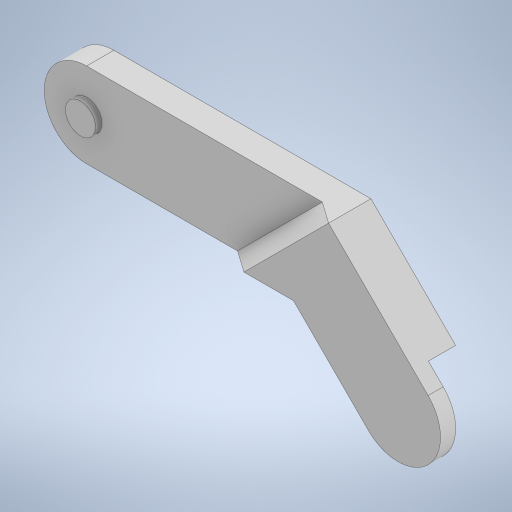
# Autodesk Inventor part: arm 1 leftt
Saved by Autodesk Inventor 2023 (Build 270158000, 158)
## iProperties
Created: 2024-06-28
Part Number: arm 1 leftt
Material: Generic
Document SubType Name: Modeling
Designer: Swoby
Density: 1 g/cm^3
Appearance: Default
Author: Swoby
Autodesk Inventor part; units mm, degrees
ref_plane "YZ Plane" through (0, 0, 0) normal (1, 0, 0) x (0, 1, 0)
ref_plane "XZ Plane" through (0, 0, 0) normal (0, 1, 0) x (-1, 0, 0)
ref_plane "XY Plane" through (0, 0, 0) normal (0, 0, 1) x (1, 0, 0)
sketch "Sketch1" plane through (0, 0, 0) normal (0, 0, 1) x (1, 0, 0)
  circle A0 centre (0, 0) radius 35
  line L0 (0, 35) -> (212.4975, 35)
  line L1 (212.4975, 35) -> (294.7487, -47.2513)
  circle A1 centre (270, -72) radius 35
  line L2 (0, -35) -> (183.5025, -35)
  line L3 (183.5025, -35) -> (245.2513, -96.7487)
  dimension "d0" = 70
  dimension "d1" = 135
  dimension "d2" = 70
  dimension "d3" = 37
  dimension "d4" = 270
  constraints: 8 end point, 4 point on circle, 4 tangent, 2 centre point, 2 horizontal, 1 coincident, 1 parallel
  measures "d0" diameter of A0
  measures "d1" angle of L0 L1
  measures "d2" diameter of A1
  measures "d3" distance from line of L2 A1.centre
  measures "d4" horizontal distance of point (0, 0) A1.centre
extrude "Extrusion1" add sketch "Sketch1" along normal blind 22.5
sketch "Sketch2" plane through (0, 0, 22.5) normal (0, 0, 1) x (1, 0, 0)
  line L0 (294.7487, -47.2513) -> (212.4975, 35) projected
  line L1 (212.4975, 35) -> (142.4975, -35)
  line L2 (0, -35) -> (183.5025, -35) projected
  arc A0 (245.2513, -96.7487) -> (294.7487, -47.2513) centre (270, -72) ccw projected
  line L3 (294.7487, -47.2513) -> (212.4975, 35) projected
  line L4 (212.4975, 35) -> (0, 35) projected
  arc A1 (0, 35) -> (0, -35) centre (0, 0) ccw projected
  line L5 (0, -35) -> (183.5025, -35) projected
  line L6 (183.5025, -35) -> (245.2513, -96.7487) projected
  line L7 (142.4975, -35) -> (183.5025, -35)
  dimension "d7" = 45
  constraints: 4 end point, 1 collinear, 1 point on line
  measures "d7" angle of L1 L2
extrude "Extrusion2" add sketch "Sketch2" along normal blind 12.5 contours A0 L6 L2 L1 L0
chamfer "Chamfer1" distance 12.5 angle 45 1 edges at (177.4975, 0, 22.5)
sketch "Sketch3" plane through (0, 0, 0) normal (0, 0, -1) x (-1, 0, 0)
  line L0 (-29, 10) -> (11, 10)
  line L1 (11, 10) -> (11, -10)
  line L2 (11, -10) -> (-29, -10)
  line L3 (-29, -10) -> (-29, 10)
  line L4 (11, 7) -> (21, 7)
  line L5 (21, 7) -> (21, -7)
  line L6 (21, -7) -> (11, -7)
  line L7 (11, -7) -> (11, 7)
  line L8 (21, 7) -> (21, 10)
  line L9 (21, 10) -> (3.9289, 27.0711)
  line L10 (16.9289, 7) -> (3.9289, 20)
  line L11 (-212.4975, 35) -> (0, 35) projected
  line L12 (3.9289, 20) -> (3.9289, 27.0711) construction
  line L13 (3.9289, 27.0711) -> (-204.5685, 27.0711)
  line L14 (3.9289, 20) -> (-197.4975, 20)
  line L15 (-212.4975, 35) -> (-142.4975, -35) construction
  line L16 (-204.5685, 27.0711) -> (-264.6396, -33)
  line L17 (-204.5685, 27.0711) -> (-130.9289, 27.0711) construction
  line L18 (-197.4975, 20) -> (-250.4975, -33)
  line L19 (-294.7487, -47.2513) -> (-212.4975, 35) projected
  line L20 (0, -35) -> (-183.5025, -35) projected
  line L21 (-264.6396, -33) -> (-250.4975, -33)
  point P0 (0, 0)
  point P1 (-194.8198, 35)
  dimension "d13" = 40
  dimension "d14" = 20
  dimension "d15" = 10
  dimension "d16" = 29
  dimension "d17" = 3
  dimension "d18" = 3
  dimension "d19" = 10
  dimension "d22" = 135
  dimension "d23" = 3
  dimension "d24" = 10
  dimension "d25" = 5
  dimension "d26" = 10
  dimension "d29" = 135
  dimension "d35" = 2
  constraints: 36 end point, 9 parallel, 4 horizontal, 3 point on line, 2 perpendicular, 1 collinear
  measures "d13" distance of L0.start L0.end
  measures "d14" distance of L0.end L1.end
  measures "d15" distance from line of L0 point (0, 0)
  measures "d16" distance from line of L3 point (0, 0)
  measures "d17" distance between parallel lines of L4 L0
  measures "d18" distance between parallel lines of L2 L6
  measures "d19" distance of L4.start L4.end
  measures "d22" angle of L8 L9
  measures "d23" distance of L4.end L8.end
  measures "d24" distance between parallel lines of L5 L1
  measures "d25" distance from line of L9 L10.start
  measures "d26" distance from line of L0 L10.end
  measures "d29" angle of L16 L17
  measures "d35" distance between parallel lines of L20 L21
sketch "Sketch4" plane through (0, 0, 0) normal (0, 0, -1) x (-1, 0, 0)
  line L0 (-142.4975, -35) -> (-183.5025, -35) projected
  line L1 (-183.5025, -35) -> (-282.4975, -35)
  line L2 (-294.7487, -47.2513) -> (-212.4975, 35) projected
  line L3 (0, -35) -> (-183.5025, -35) projected
  arc A0 (-294.7487, -47.2513) -> (-245.2513, -96.7487) centre (-270, -72) ccw projected
  line L4 (-183.5025, -35) -> (-245.2513, -96.7487) projected
  line L5 (0, -35) -> (-183.5025, -35) projected
  arc A1 (0, -35) -> (0, 35) centre (0, 0) ccw projected
  line L6 (-212.4975, 35) -> (0, 35) projected
  line L7 (-294.7487, -47.2513) -> (-212.4975, 35) projected
  line L8 (-282.4975, -35) -> (-294.7487, -47.2513)
  constraints: 4 end point, 2 collinear, 1 point on line
extrude "Extrusion3" cut sketch "Sketch4" against normal blind 22.5 contours L4 A0 L2 L1
extrude "Extrusion4" cut sketch "Sketch3" against normal blind 20
sketch "Sketch5" plane through (0, 0, 22.5) normal (0, 0, 1) x (1, 0, 0)
  circle A0 centre (0, 0) radius 12.5
  dimension "d30" = 25
  constraints: 1 centre point, 1 coincident
  measures "d30" diameter of A0
extrude "Extrusion5" add sketch "Sketch5" along normal blind 5
sketch "Sketch6" plane through (0, 0, 20) normal (0, 0, -1) x (-1, 0, 0)
  line L0 (11, 7) -> (16.9289, 7) projected
  line L1 (11, 10) -> (11, 7) projected
  line L2 (-29, 10) -> (11, 10) projected
  line L3 (-29, -10) -> (-29, 10) projected
  line L4 (11, -10) -> (-29, -10) projected
  line L5 (11, -7) -> (11, -10) projected
  line L6 (21, -7) -> (11, -7) projected
  line L7 (21, 10) -> (21, -7) projected
  line L8 (3.9289, 27.0711) -> (21, 10) projected
  line L9 (-204.5685, 27.0711) -> (3.9289, 27.0711) projected
  line L10 (-264.6396, -33) -> (-204.5685, 27.0711) projected
  line L11 (-250.4975, -33) -> (-264.6396, -33) projected
  line L12 (-197.4975, 20) -> (-250.4975, -33) projected
  line L13 (3.9289, 20) -> (-197.4975, 20) projected
  line L14 (16.9289, 7) -> (3.9289, 20) projected
  line L15 (-264.6396, -33) -> (-204.5685, 27.0711) projected
  line L16 (-254.6396, -23) -> (-240.4975, -23)
  line L17 (-197.4975, 20) -> (-250.4975, -33) projected
  point P0 (0, 0)
  dimension "d36" = 10
  constraints: 2 end point, 2 point on line, 1 horizontal
  measures "d36" distance between parallel lines of L11 L16
extrude "Extrusion6" cut sketch "Sketch6" against normal up to surface (2.5 mm away) contours L12 L11 L10 L16
sketch "Sketch7" plane through (0, 0, 22.5) normal (0, 0, -1) x (-1, 0, 0)
  line L0 (-254.6396, -23) -> (-240.4975, -23) projected
  line L1 (-264.6396, -33) -> (-254.6396, -23) projected
  line L2 (-250.4975, -33) -> (-264.6396, -33) projected
  line L3 (-240.4975, -23) -> (-250.4975, -33) projected
  line L4 (-264.6396, -33) -> (-280, -48.3604)
  line L5 (-280, -48.3604) -> (-265.8579, -48.3604)
  line L6 (-265.8579, -48.3604) -> (-250.4975, -33)
  point P0 (0, 0)
  constraints: 6 end point, 2 collinear, 1 parallel
extrude "Extrusion7" cut sketch "Sketch7" against normal blind 10
body "Solid1"
